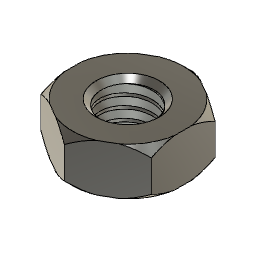
M4-70 Nut v2 (Autodesk Fusion 360 design; units mm, degrees)
Autodesk Fusion 360 part; units mm, degrees
sketch "Sketch1" plane through (0, 0, 0) normal (0, 0, 1) x (1, 0, 0)
  line L0 (3.5, 2.0207) -> (0, 4.0415)
  line L1 (0, 4.0415) -> (-3.5, 2.0207)
  line L2 (-3.5, 2.0207) -> (-3.5, -2.0207)
  line L3 (-3.5, -2.0207) -> (0, -4.0415)
  line L4 (0, -4.0415) -> (3.5, -2.0207)
  line L5 (3.5, -2.0207) -> (3.5, 2.0207)
  dimension "d1" = 7
  measures "d1" distance of L2 L5
extrude "Extrude1" add sketch "Sketch1" along normal blind 3
sketch "Sketch5" plane through (0, 0, 0) normal (1, 0, 0) x (0, 1, 0)
  line L0 (2.0207, 3) -> (4.0415, 3)
  line L1 (4.0415, 3) -> (3.5415, 3)
  line L2 (4.0415, 3) -> (4.0415, 2.5)
  line L3 (4.0415, 2.5) -> (3.5415, 3)
  point P0 (4.0415, 3)
  dimension "d4" = 0.5
  dimension "d5" = 0.5
  constraint coincident P0 L0.end
  constraint parallel L0 L1
  constraint perpendicular L0 L2
  measures "d4" distance of P0 L1.end
  measures "d5" distance of P0 L2.end
revolve "Revolve1" cut sketch "Sketch5" angle 360 about axis through (0, 0, 1.75) along (0, 0, 1)
ref_plane "WorkPlane1" through (0, 0, 1.5) normal (0, 0, 1) x (1, 0, 0)
mirror "Mirror1" about plane through (0, 0, 1.5) normal (0, 0, 1) of "Revolve1"
hole "Hole1" at (0.0059, -0.0199, 3) direction (0, 0, -1) diameter 3.332 depth 3 tip angle 180 countersink diameter 4 countersink angle 90
thread "Thread1" "GB Metric profile 4.0 M4x0.7 6H" major diameter 4.1095 minor diameter 3.332 pitch 0.7 angle 60 modelled right hand crest width 0.193 on face at (0.089, -1.6839, 1.7773) crest through (1.6719, -0.0199, 2.491)
